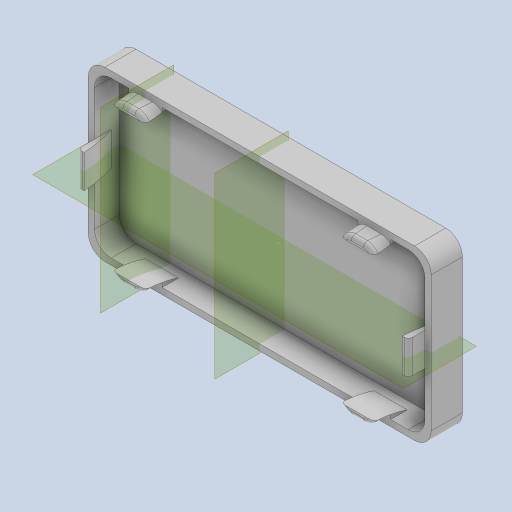
# Autodesk Inventor part: caja_inferior
Saved by Autodesk Inventor 2024 (Build 280153000, 153)
## iProperties
Created: 2025-12-14
Part Number: caja_inferior
Material: Genérico
Document SubType Name: Modeling
Designer: ANDRES
Density: 1 g/cm^3
Appearance: Valor por defecto
Author: ANDRES
Autodesk Inventor part; units mm, degrees
ref_plane "YZ Plane" through (0, 0, 0) normal (1, 0, 0) x (0, 1, 0)
ref_plane "XZ Plane" through (0, 0, 0) normal (0, 1, 0) x (-1, 0, 0)
ref_plane "XY Plane" through (0, 0, 0) normal (0, 0, 1) x (1, 0, 0)
sketch "Boceto1" plane through (0, 0, 0) normal (0, 0, 1) x (1, 0, 0)
  line L0 (-39.75, 21.75) -> (42.75, 21.75)
  line L1 (42.75, 21.75) -> (42.75, -18.75)
  line L2 (42.75, -18.75) -> (-39.75, -18.75)
  line L3 (-39.75, -18.75) -> (-39.75, 21.75)
  dimension "ancho" = 40.5
  dimension "largo" = 82.5
  constraints: 8 end point, 2 parallel, 1 horizontal, 1 perpendicular
  measures "ancho" distance of L0.end L1.end
  measures "largo" distance between parallel lines of L3 L1
extrude "Extrusión1" add sketch "Boceto1" along normal blind 1.5
sketch "Boceto2" plane through (0, 0, 1.5) normal (0, 0, 1) x (1, 0, 0)
  line L0 (-39.75, -18.75) -> (-39.75, 21.75) projected
  line L1 (-39.75, 21.75) -> (42.75, 21.75) projected
  line L2 (42.75, 21.75) -> (42.75, -18.75) projected
  line L3 (42.75, -18.75) -> (-39.75, -18.75) projected
  line L4 (41.25, 20.25) -> (-38.25, 20.25)
  line L5 (-38.25, 20.25) -> (-38.25, -17.25)
  line L6 (-38.25, -17.25) -> (41.25, -17.25)
  line L7 (41.25, -17.25) -> (41.25, 20.25)
  point P0 (0, 0)
  dimension "d5" = 1.5
  constraints: 8 end point, 3 other
  measures "d5" distance between parallel lines of L1 L4
extrude "Extrusión2" add sketch "Boceto2" along normal blind 6
sketch "Boceto3" plane through (42.75, -18.75, 0) normal (1, 0, 0) x (0, 0, -1)
  line L0 (-11, 26.75) -> (-2, 26.75)
  line L1 (-2, 26.75) -> (-2, 12.75)
  line L2 (-2, 12.75) -> (-11, 12.75)
  line L3 (-11, 12.75) -> (-11, 26.75)
  line L4 (-11, 26.75) -> (-2, 12.75) construction
  line L5 (-2, 26.75) -> (-11, 12.75) construction
  line L6 (0, 40.5) -> (-7.5, 40.5) projected
  line L7 (0, 0) -> (-7.5, 0) projected
  point P0 (0, 18.75)
  point P1 (-6.5, 19.75)
  point P2 (-6.5, 12.75)
  dimension "d8" = 14
  dimension "d9" = 9
  dimension "d10" = 20.75
  dimension "d11" = 13.75
  dimension "d12" = 12.75
  dimension "d13" = 2
  constraints: 12 end point, 3 midpoint, 2 parallel, 1 horizontal, 1 perpendicular
  measures "d8" distance between parallel lines of L2 L0
  measures "d9" distance between parallel lines of L1 L3
  measures "d10" distance from line of L6 point (-6.5, 19.75)
  measures "d11" distance between parallel lines of L6 L0
  measures "d12" distance from line of L7 point (-6.5, 12.75)
  measures "d13" distance from line of point (0, 18.75) L1
extrude "Extrusión3" [suppressed]
fillet "Empalme1" [suppressed]
ref_plane "Plano de trabajo1" through (1.5, -17.25, 1.5) normal (-1, 0, 0) x (0, 0, 1)
ref_plane "Plano de trabajo2" through (-38.25, 1.5, 1.5) normal (0, -1, 0) x (1, 0, 0)
sketch "Boceto4" plane through (41.25, -17.25, 1.5) normal (-1, 0, 0) x (0, 0, 1)
  line L0 (0, 0) -> (6, 0) projected
  line L1 (6, 37.5) -> (6, 0) projected
  line L2 (6, 37.5) -> (0, 37.5) projected
  line L3 (0, 0) -> (0, 37.5) projected
  line L4 (6, 0) -> (6, -1.5) projected
  line L5 (6, -1.5) -> (-1.5, -1.5) projected
  line L6 (-1.5, -1.5) -> (-1.5, 39) projected
  line L7 (-1.5, 39) -> (6, 39) projected
  line L8 (6, 39) -> (6, 37.5) projected
  line L9 (10, 37.5) -> (2, 37.5)
  arc A0 (2, 37.5) -> (10, 36) centre (11.4775, 65.9636) ccw
  line L10 (10, 37.5) -> (10, 36)
  point P0 (-1.5, 17.25)
  point P1 (11.479, 40.458)
  point P2 (2, 37.5)
  dimension "d24" = 8
  dimension "d25" = 30
  dimension "d26" = 1.5
  constraints: 4 end point, 2 point on circle, 1 centre point, 1 coincident, 1 horizontal, 1 horizontal alignment, 1 midpoint, 1 vertical
  measures "d24" distance of L9.start L9.end
  measures "d25" radius of A0
  measures "d26" distance of L9.start L10.end
extrude "Extrusión4" [suppressed]
fillet "Empalme2" [suppressed]
mirror "Simetría1" [suppressed]
mirror "Simetría2" [suppressed]
fillet "Empalme3" radius 4 8 edges at (41.25, -17.25, 4.5) (41.25, 20.25, 4.5) (-38.25, 20.25, 4.5) (-38.25, -17.25, 4.5) (-39.75, -18.75, 3.75) (42.75, -18.75, 3.75) (42.75, 21.75, 3.75) (-39.75, 21.75, 3.75)
sketch "Boceto5" plane through (0, 0, 1.5) normal (0, 0, 1) x (1, 0, 0)
  point P0 (0, 0)
sketch "Boceto6" plane through (1.5, -17.25, 1.5) normal (-1, 0, 0) x (0, 0, 1)
  line L0 (6, 0) -> (6, -1.5) projected
  line L1 (6, -1.5) -> (-1.5, -1.5) projected
  line L2 (-1.5, -1.5) -> (-1.5, 39) projected
  line L3 (-1.5, 39) -> (6, 39) projected
  line L4 (6, 39) -> (6, 37.5) projected
  line L5 (6, 37.5) -> (0, 37.5) projected
  line L6 (0, 37.5) -> (0, 0) projected
  line L7 (0, 0) -> (6, 0) projected
  line L8 (2, 37.5) -> (10, 37.5)
  line L9 (10, 37.5) -> (10, 36)
  arc A0 (2, 37.5) -> (10, 36) centre (11.4775, 65.9636) ccw
  point P0 (-1.5, 17.25)
  point P1 (2, 37.5)
  dimension "d31" = 1.5
  dimension "d32" = 8
  dimension "d33" = 30
  constraints: 4 end point, 2 coincident, 2 point on circle, 1 centre point, 1 horizontal, 1 midpoint, 1 vertical
  measures "d31" distance of L8.end L9.end
  measures "d32" distance of L8.start L8.end
  measures "d33" radius of A0
extrude "Extrusión5" [suppressed]
fillet "Empalme4" [suppressed]
fillet "Empalme5" [suppressed]
mirror "Simetría3" [suppressed]
sketch "Boceto7" plane through (-38.25, 1.5, 1.5) normal (0, -1, 0) x (1, 0, 0)
  line L0 (79.5, 0) -> (79.5, 6) projected
  line L1 (81, 6) -> (81, -1.5) projected
  line L2 (81, -1.5) -> (-1.5, -1.5) projected
  line L3 (-1.5, -1.5) -> (-1.5, 6) projected
  line L4 (-1.5, 6) -> (0, 6) projected
  line L5 (0, 6) -> (0, 0) projected
  line L6 (0, 0) -> (79.5, 0) projected
  line L7 (79.5, 2) -> (79.5, 10)
  line L8 (79.5, 10) -> (78, 10)
  arc A0 (78, 10) -> (79.5, 2) centre (107.9636, 11.4775) ccw
  line L9 (79.5, 6) -> (81, 6) projected
  point P0 (38.25, -1.5)
  point P1 (79.5, 6)
  point P2 (79.5, 6)
  dimension "d38" = 1.5
  dimension "d39" = 8
  dimension "d40" = 30
  constraints: 4 end point, 2 coincident, 2 point on circle, 1 centre point, 1 midpoint, 1 perpendicular, 1 vertical
  measures "d38" distance of L7.end L8.end
  measures "d39" distance of L7.start L7.end
  measures "d40" radius of A0
extrude "Extrusión6" add sketch "Boceto7" along normal mid plane 8 contours A0 L8 L7 L0
fillet "Empalme6" [suppressed]
fillet "Empalme7" radius 1 1 edges at (41.25, 1.5, 11.5)
mirror "Simetría4" about plane through (1.5, -17.25, 1.5) normal (-1, 0, 0) of "Extrusión6", "Empalme7"
ref_plane "Plano de trabajo3" through (-26, -17.25, 1.5) normal (-1, 0, 0) x (0, 0, 1)
sketch "Boceto8" plane through (-26, -17.25, 1.5) normal (-1, 0, 0) x (0, 0, 1)
  line L0 (16, -14.3135) -> (16, -15.8135)
  line L1 (16, -15.8135) -> (-1.5, -15.8135)
  line L2 (-1.5, -15.8135) -> (-1.5, 39)
  line L3 (-1.5, 39) -> (6, 39)
  line L4 (6, 39) -> (6, 37.5)
  line L5 (6, 37.5) -> (0, 37.5)
  line L6 (0, 37.5) -> (0, -14.3135)
  line L7 (0, -14.3135) -> (16, -14.3135)
  line L8 (2, 37.5) -> (10, 37.5)
  line L9 (10, 37.5) -> (10, 36)
  arc A0 (2, 37.5) -> (10, 36) centre (11.4775, 65.9636) ccw
  line L10 (-1.5, 39) -> (6, 39) projected
  line L11 (6, 39) -> (6, 37.5) projected
  line L12 (6, 37.5) -> (0, 37.5) projected
  line L13 (0, 37.5) -> (0, 0) projected
  line L14 (0, 0) -> (6, 0) projected
  line L15 (6, 0) -> (6, -1.5) projected
  line L16 (6, -1.5) -> (-1.5, -1.5) projected
  line L17 (-1.5, -1.5) -> (-1.5, 39) projected
  point P0 (-1.5, 17.25)
  point P1 (25.1174, 2.4365)
  point P2 (42.6174, 22.1865)
  point P3 (38.6174, 22.1865)
  point P4 (2, 37.5)
  dimension "d46" = 1.5
  dimension "d47" = 8
  dimension "d48" = 30
  constraints: 18 end point, 2 coincident, 2 point on circle, 1 centre point, 1 horizontal, 1 midpoint, 1 vertical, 3 other
  measures "d46" distance of L8.end L9.end
  measures "d47" distance of L8.start L8.end
  measures "d48" radius of A0
extrude "Extrusión7" add sketch "Boceto8" along normal mid plane 8 contours L5 L8 L9 A0
fillet "Empalme8" radius 3 2 edges at (-22, 20.25, 9.5) (-30, 20.25, 9.5)
fillet "Empalme9" radius 1 3 edges at (-23.0987, 19.8482, 11.5) (-28.9013, 19.8482, 11.5) (-26, 20.25, 11.5)
mirror "Simetría5" about plane through (-38.25, 1.5, 1.5) normal (0, -1, 0) of "Extrusión7", "Empalme9", "Empalme8"
mirror "Simetría6" about plane through (1.5, -17.25, 1.5) normal (-1, 0, 0) of "Extrusión7", "Empalme9", "Empalme8", "Simetría5"
equation "\"d5\" = espesor"
equation "\"d26\" = espesor"
equation "\"d31\" = espesor"
equation "\"d38\" = espesor"
equation "\"d46\" = d49"
equation "\"d17\" = 0.5 * largo - espesor"
equation "\"d18\" = 0.5 * ancho - espesor"
equation "\"d45\" = 0.333333 * largo"
equation "\"espesor\" = 1.5"
equation "\"d49\" = 1.5"
